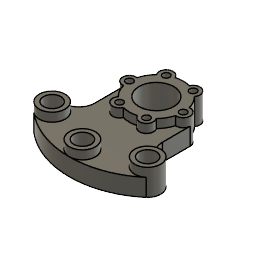
complex drawing (Autodesk Fusion 360 design; units mm, degrees)
part number: 2026-08-21-00-05-20-576
Autodesk Fusion 360 part; units mm, degrees
sketch "Sketch1" plane through (0, 0, 0) normal (0, 1, 0) x (1, 0, 0)
  line L0 (-50, 0) -> (50, 0) construction
  line L1 (0, 105.7095) -> (0, -105.7095) construction
  line L2 (-55, -65) -> (55, -65) construction
  circle A0 centre (-55, -65) radius 15
  circle A1 centre (-55, -65) radius 15
  circle A2 centre (55, -65) radius 15
  circle A3 centre (-55, -65) radius 10
  circle A4 centre (55, -65) radius 10
  circle A5 centre (0, 0) radius 20
  circle A6 centre (31, 0) radius 4
  circle A7 centre (-31, 0) radius 4
  line L3 (0, 0) -> (44, 0) construction
  circle A8 centre (-15.5, -26.8468) radius 4
  circle A9 centre (15.5, 26.8468) radius 4
  line L4 (0, 0) -> (45, 0) construction
  line L5 (0, 0) -> (44, 0) construction
  circle A10 centre (15.5, -26.8468) radius 4
  circle A11 centre (-15.5, 26.8468) radius 4
  arc A12 (-29.9677, 7.9331) -> (-29.9677, -7.9331) centre (-31, 0) ccw
  arc A13 (-8.1136, 29.9194) -> (-21.8542, 21.9863) centre (-15.5, 26.8468) ccw
  arc A14 (-21.8542, 21.9863) -> (-29.9677, 7.9331) centre (0, 0) ccw
  arc A15 (21.8542, 21.9863) -> (8.1136, 29.9194) centre (15.5, 26.8468) ccw
  arc A16 (8.1136, 29.9194) -> (-8.1136, 29.9194) centre (0, 0) ccw
  arc A17 (29.9677, -7.9331) -> (29.9677, 7.9331) centre (31, 0) ccw
  arc A18 (29.9677, 7.9331) -> (21.8542, 21.9863) centre (0, 0) ccw
  arc A19 (8.1136, -29.9194) -> (21.8542, -21.9863) centre (15.5, -26.8468) ccw
  arc A20 (-21.8542, -21.9863) -> (-8.1136, -29.9194) centre (-15.5, -26.8468) ccw
  arc A21 (-29.9677, -7.9331) -> (-21.8542, -21.9863) centre (0, 0) ccw
  arc A22 (-8.1136, -29.9194) -> (8.1136, -29.9194) centre (0, 0) ccw
  arc A23 (21.8542, -21.9863) -> (29.9677, -7.9331) centre (0, 0) ccw
  line L6 (39, 0) -> (39, -32.0607)
  arc A24 (-64.7059, -76.4366) -> (64.7059, -76.4366) centre (0, -0.1926) ccw
  circle A25 centre (0, -85.1926) radius 15
  circle A26 centre (0, -85.1926) radius 10
  arc A27 (39, -32.0607) -> (55.9091, -50.0276) centre (57, -32.0607) ccw
  arc A28 (-55.9091, -50.0276) -> (-39, -32.0607) centre (-57, -32.0607) ccw
  line L7 (-39, 0) -> (-39, -32.0607)
  point P0 (0, -65)
  dimension "d1" = 100
  dimension "d2" = 65
  dimension "d3" = 110
  dimension "d4" = 30
  dimension "d5" = 30
  dimension "d6" = 30
  dimension "d7" = 20
  dimension "d8" = 20
  dimension "d11" = 8
  dimension "d12" = 16
  dimension "d21" = 105.7095
  dimension "d22" = 200
  dimension "d23" = 30
  dimension "d24" = 20
  dimension "d25" = 36
  dimension "d26" = 8
  dimension "d27" = 8
  dimension "d28" = 8
  dimension "d29" = 40
  dimension "d30" = 8
  dimension "d31" = 8
  dimension "d32" = 8
  dimension "d33" = 31
  dimension "d34" = 8
  dimension "d35" = 8
  constraint midpoint L0 A5.centre
  constraint coincident A5.centre L3.start
  constraint horizontal L0
  constraint midpoint L1 A5.centre
  constraint perpendicular L0 L1
  constraint midpoint L2 P0
  constraint coincident L1 P0
  constraint perpendicular L1 L2
  constraint coincident L2.start A0.centre
  constraint coincident L2.end A2.centre
  constraint concentric A0 A3
  constraint concentric A2 A4
  constraint concentric A6 A17
  constraint symmetric L1 A6 A7
  constraint symmetric L1 A12 A17
  constraint horizontal L3
  constraint horizontal L4
  constraint horizontal L5
  constraint concentric A16 A18
  constraint concentric A21 A22
  constraint concentric A22 A23
  constraint coincident L4 L6.start
  constraint coincident L1 A24.centre
  constraint tangent A2 A24
  constraint coincident A0 A24.start
  constraint coincident A2 A24.end
  constraint coincident L1 A25.centre
  constraint concentric A25 A26
  constraint tangent A24 A25
  constraint tangent A2 A27
  constraint tangent L6 A27
  constraint coincident A2 A27.end
  constraint symmetric L1 L6.start L7.start
  constraint symmetric L1 L6.end A28.end
  constraint symmetric L1 A27.end A28.start
  constraint symmetric L1 A27 A28
  measures "d1" distance of L0.start L0.end
  measures "d2" distance of L0 L2
  measures "d3" distance of L2.start L2.end
  measures "d4" diameter of A0
  measures "d5" diameter of A1
  measures "d6" diameter of A2
  measures "d7" diameter of A3
  measures "d8" diameter of A4
  measures "d11" diameter of A6
  measures "d12" diameter of A17
  measures "d21" distance of L1.end A5.centre
  measures "d22" diameter of A24
  measures "d23" diameter of A25
  measures "d24" diameter of A26
  measures "d25" diameter of A27
  measures "d26" radius of A19
  measures "d27" diameter of A10
  measures "d28" diameter of A8
  measures "d29" diameter of A5
  measures "d30" diameter of A9
  measures "d31" diameter of A11
  measures "d32" radius of A13
  measures "d33" radius of A14
  measures "d34" diameter of A8
  measures "d35" radius of A15
extrude "Extrude1" add sketch "Sketch1" along normal blind 20 contours A0 A1 A2 A12 A17 A19 A20 A21 A22 A23 L6 A24 A27 A28 L7 makes body 1
extrude "Extrude2" add sketch "Sketch1" along normal blind 30 separate body contours A0 A1 | A12 A13 A14 A15 A16 A17 A18 A19 A20 A21 A22 A23 | A2 makes body 2 at (-40.0745, 10, 66.4935) makes body 3 at (69.9255, 10, 66.4935) makes body 4 at (19.9751, 10, 0.9969)
extrude "Extrude3" add sketch "Sketch1" along normal blind 30 contours A25 bodies 1
combine "Combine1" operation add target body 1 tool bodies 4 2 3
